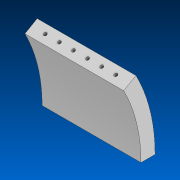
# Autodesk Inventor part: HoodBrace
Saved by Autodesk Inventor 2022.2 (Build 262287000, 287)
## iProperties
Created: 2022-04-24
Part Number: HoodBrace
Material: Generic
Document SubType Name: Modeling
Designer: omard
Density: 1 g/cm^3
Appearance: Default
Author: omard
Autodesk Inventor part; units mm, degrees
ref_plane "YZ Plane" through (0, 0, 0) normal (1, 0, 0) x (0, 1, 0)
ref_plane "XZ Plane" through (0, 0, 0) normal (0, 1, 0) x (-1, 0, 0)
ref_plane "XY Plane" through (0, 0, 0) normal (0, 0, 1) x (1, 0, 0)
sketch "Sketch1" plane through (0, 0, 0) normal (1, 0, 0) x (0, 1, 0)
  arc A0 (0, -277.0467) -> (138.5234, -239.9295) centre (0, 0) ccw
  arc A1 (0, -302.4467) -> (151.2234, -261.9266) centre (0, 0) ccw
  line L0 (138.5234, -239.9295) -> (151.2234, -261.9266)
  line L1 (0, -277.0467) -> (0, -302.4467)
  line L2 (127.3792, -246.0273) -> (140.2248, -268.2766)
  line L3 (140.2248, -268.2766) -> (162.2219, -255.5766)
  line L4 (162.2219, -255.5766) -> (149.5219, -233.5795)
  line L5 (149.5219, -233.5795) -> (127.5248, -246.2795)
  line L6 (127.5248, -246.2795) -> (162.2219, -255.5766) construction
  line L7 (140.2248, -268.2766) -> (149.5219, -233.5795) construction
  point P0 (144.8734, -250.928)
  point P1 (140.0915, -268.0455)
  dimension "d1" = 277.0467
  dimension "d2" = 30
  dimension "d4" = 25.4
  dimension "d5" = 25.4
  constraints: 16 end point, 5 point on circle, 4 midpoint, 3 parallel, 3 point on line, 2 centre point, 2 coincident, 1 line through centre, 1 perpendicular, 1 vertical
  measures "d1" radius of A0
  measures "d2" angle of L1 L0
  measures "d4" distance of L3.end L2.end
  measures "d5" distance of L1.start L1.end
extrude "Extrusion1" add sketch "Sketch1" along normal mid plane 177.8 contours A0 L2 A1 L1
sketch "Sketch2" plane through (-88.9, 0, -302.4467) normal (0, -1, 0) x (1, 0, 0)
  line L0 (177.8, 0) -> (0, 0) projected
  line L1 (177.8, 25.4) -> (177.8, 0) projected
  point P0 (88.9, 302.4467)
  point P1 (165.1, 12.7)
  dimension "d8" = 12.7
  dimension "d9" = 12.7
  measures "d8" distance from line of L0 point (165.1, 12.7)
  measures "d9" distance from line of L1 point (165.1, 12.7)
hole "Hole1" at (76.2, 0, -289.7467) direction (0, 1, 0) diameter 4.445 depth 38.1 start extended yes counterbore diameter 5.588 counterbore depth 8.255
sketch "Sketch3" plane through (-88.9, 127.3792, -246.0273) normal (0, 0.8660254, 0.5) x (1, 0, 0)
  line L0 (88.9, 0) -> (88.9, 25.6912) projected
  line L1 (177.8, 25.4245) -> (177.8, 0) projected
  point P0 (88.9, -276.7555)
  point P1 (152.4, 12.9912)
  dimension "d17" = 25.4
  dimension "d18" = 12.7
  measures "d17" distance from line of point (152.4, 12.991) L1
  measures "d18" vertical distance of L0.end point (152.4, 12.991)
hole "Hole2" at (63.5, 133.8748, -257.278) direction (0, -0.8660254, -0.5) diameter 4.445 depth 38.1 start extended yes counterbore diameter 5.588 counterbore depth 8.255
pattern_linear "Rectangular Pattern1" count 7 spacing 25.4 along (-1, 0, 0) of "Hole1"
pattern_linear "Rectangular Pattern2" count 6 spacing 25.4 along (-1, 0, 0) of "Hole2"
body "Solid1"
